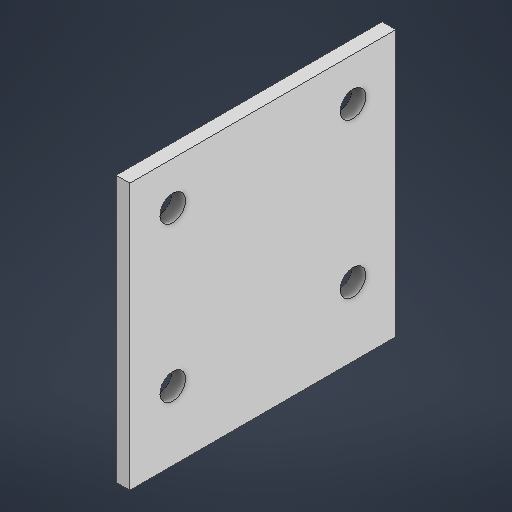
# Autodesk Inventor part: Bracket_side
Saved by Autodesk Inventor 2026.1 (Build 301233020, 233B)
## iProperties
Created: 2025-10-11
Part Number: Bracket_side
Material: Generic
Document SubType Name: Modeling
Designer: Alexander
Density: 1 g/cm^3
Appearance: Default
Author: Alexander
Autodesk Inventor part; units mm, degrees
ref_plane "YZ Plane" through (0, 0, 0) normal (1, 0, 0) x (0, 1, 0)
ref_plane "XZ Plane" through (0, 0, 0) normal (0, 1, 0) x (-1, 0, 0)
ref_plane "XY Plane" through (0, 0, 0) normal (0, 0, 1) x (1, 0, 0)
sketch "Sketch1" plane through (0, 0, 0) normal (1, 0, 0) x (0, 1, 0)
  line L0 (77.5, 77.5) -> (-77.5, 77.5)
  line L1 (-77.5, 77.5) -> (-77.5, -77.5)
  line L2 (-77.5, -77.5) -> (77.5, -77.5)
  line L3 (77.5, -77.5) -> (77.5, 77.5)
  circle A0 centre (52.5, 52.5) radius 7.5
  circle A1 centre (52.5, -52.5) radius 7.5
  circle A2 centre (-37.5, 52.5) radius 7.5
  circle A3 centre (-37.5, -52.5) radius 7.5
  point P0 (0, 0)
  point P1 (0, -77.5)
  point P2 (-77.5, 0)
  dimension "d0" = 155
  dimension "d1" = 155
  dimension "d2" = 25
  dimension "d3" = 25
  dimension "d4" = 15
  dimension "d7" = 105
  dimension "d10" = 90
  constraints: 8 end point, 4 centre point, 2 horizontal, 2 midpoint, 2 parallel, 1 coincident, 1 horizontal alignment, 1 perpendicular, 1 vertical, 1 vertical alignment, 6 other
  measures "d0" distance of L2.end L1.end
  measures "d1" distance of L1.end L0.end
  measures "d2" horizontal distance of L0.start point (52.5, 52.5)
  measures "d3" horizontal distance of L0.start point (52.5, 52.5)
  measures "d4" diameter of A0
  measures "d7" distance of A0.centre A1.centre
  measures "d10" distance of A0.centre A2.centre
extrude "Extrusion1" add sketch "Sketch1" along normal mid plane 8
body "Solid1"
